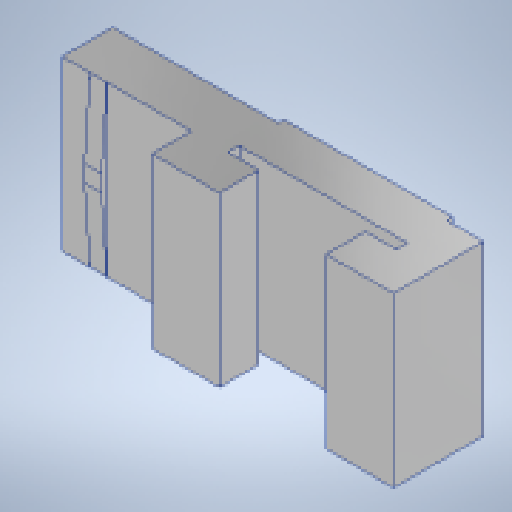
# Autodesk Inventor part: KatzeFEM
Saved by Autodesk Inventor 2025 (Build 290162010, 162A)
## iProperties
Created: 2025-02-05
Part Number: KatzeFEM
Material: Aluminium 6061, Katze
Document SubType Name: Modeling
Designer: Admin
Density: 2.7 g/cm^3
Appearance: Aluminium - flach(1)
Mass: 59.0207 g
Surface Area: 77.2722 cm^2
Volume: 21.8595 cm^3
Author: Admin
Autodesk Inventor part; units mm, degrees
ref_plane "YZ Plane" through (0, 0, 0) normal (1, 0, 0) x (0, 1, 0)
ref_plane "XZ Plane" through (0, 0, 0) normal (0, 1, 0) x (-1, 0, 0)
ref_plane "XY Plane" through (0, 0, 0) normal (0, 0, 1) x (1, 0, 0)
sketch "Skizze1" plane through (0, 0, 0) normal (0, 0, 1) x (1, 0, 0)
  line L0 (-41.25, -314) -> (-33.75, -314) projected
  line L1 (-41.25, -312) -> (-41.25, -314) projected
  line L2 (-11.25, -312) -> (-41.25, -312) projected
  line L3 (-18.75, -314) -> (-11.25, -314) projected
  line L4 (-11.25, -314) -> (-11.25, -312) projected
  line L5 (-18.75, -314) -> (-16.75, -314)
  line L6 (-16.75, -314) -> (-16.75, -321)
  line L7 (-16.75, -321) -> (-4.75, -321)
  line L8 (-4.75, -321) -> (-4.75, -305)
  line L9 (-4.75, -305) -> (-70.75, -305)
  line L10 (-70.75, -305) -> (-70.75, -314)
  line L11 (-47.75, -314) -> (-47.75, -321)
  line L12 (-47.75, -321) -> (-35.75, -321)
  line L13 (-35.75, -321) -> (-35.75, -314)
  line L14 (-35.75, -314) -> (-33.75, -314)
  line L15 (-70.75, -314) -> (-65.75, -314)
  line L16 (-65.75, -314) -> (-65.75, -315)
  line L17 (-65.75, -315) -> (-62.75, -315)
  line L18 (-62.75, -315) -> (-62.75, -314)
  line L19 (-62.75, -314) -> (-47.75, -314)
  line L20 (-23.75, -312) -> (-23.75, -311)
  line L21 (-23.75, -311) -> (-26.25, -311)
  line L22 (-26.25, -311) -> (-28.75, -311)
  line L23 (-28.75, -311) -> (-28.75, -312)
  line L24 (-26.25, -311) -> (-26.25, -312) construction
  point P0 (0, 0)
  point P1 (-64.25, -315)
  dimension "d0" = 2
  dimension "d1" = 7
  dimension "d2" = 12
  dimension "d3" = 16
  dimension "d4" = 12
  dimension "d5" = 2
  dimension "d6" = 3
  dimension "d7" = 38
  dimension "d8" = 5
  dimension "d9" = 1
  dimension "d20" = 1
  dimension "d21" = 5
  constraints: 40 end point, 15 perpendicular, 9 point on line, 2 midpoint, 1 collinear, 1 horizontal, 1 vertical
  measures "d0" distance of L3.start L5.end
  measures "d1" distance of L5.end L6.end
  measures "d2" distance of L6.end L7.end
  measures "d3" distance of L7.end L8.end
  measures "d4" distance of L11.end L12.end
  measures "d5" distance of L0.end L13.end
  measures "d6" distance of L16.end L17.end
  measures "d7" horizontal distance of L24.end point (-64.25, -315)
  measures "d8" distance of L10.end L15.end
  measures "d9" distance of L17.end L18.end
  measures "d20" distance of L20.start L20.end
  measures "d21" distance of L22.end L20.end
extrude "Extrusion1" add sketch "Skizze1" along normal blind 30 contours L0 L13 L12 L11 L19 L18 L17 L16 L15 L10 L9 L8 L7 L6 L3 L4 L2 L20 L21 L22 L23 L1
chamfer "Fasen1" distance 1 distance2 13.5 1 edges at (-64.25, -315, 30) measured on face at (-64.25, -314.5, 30)
chamfer "Fasen2" distance 1 distance2 13.5 1 edges at (-64.25, -315, 0) measured on face at (-64.25, -314.5, 0)
sketch "Skizze2" plane through (-70.75, -305, 0) normal (0, 1, 0) x (1, 0, 0)
  line L0 (29.5, 0) -> (59.5, 0) projected
  line L1 (59.5, 0) -> (59.5, -30) projected
  line L2 (29.5, 0) -> (59.5, 0)
  line L3 (59.5, 0) -> (59.5, -30)
  line L4 (59.5, -30) -> (29.5, -30)
  line L5 (29.5, -30) -> (29.5, 0)
  point P0 (70.75, 0)
  constraints: 8 end point, 2 parallel, 1 horizontal, 1 perpendicular
extrude "Extrusion2" add sketch "Skizze2" along normal blind 1
